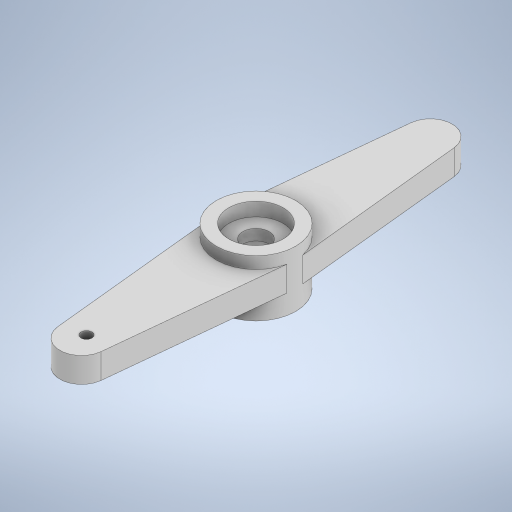
# Autodesk Inventor part: Servo_small_top
Saved by Autodesk Inventor 2023 (Build 270158000, 158)
## iProperties
Created: 2024-07-03
Part Number: Servo_small_top
Material: Generic
Document SubType Name: Modeling
Designer: Swoby
Density: 1 g/cm^3
Appearance: Default
Author: Swoby
Autodesk Inventor part; units mm, degrees
ref_plane "YZ Plane" through (0, 0, 0) normal (1, 0, 0) x (0, 1, 0)
sketch "Sketch1" plane through (0, 0, 0) normal (0, 1, 0) x (-1, 0, 0)
  circle A0 centre (0, 0) radius 2.5
  circle A1 centre (0, 0) radius 3.65
  dimension "d0" = 5
  dimension "d1" = 7.3
  constraints: 2 centre point, 2 coincident
  measures "d0" diameter of A0
  measures "d1" diameter of A1
extrude "Extrusion1" add sketch "Sketch1" along normal blind 5.2
ref_plane "Work Plane1" through (0, 3.95, 0) normal (0, 1, 0) x (1, 0, 0)
sketch "Sketch2" plane through (0, 3.95, 0) normal (0, 1, 0) x (1, 0, 0)
  circle A0 centre (0, 0) radius 2.5 projected
  circle A1 centre (0, 0) radius 1.2
  dimension "d5" = 2.4
  constraints: 1 centre point, 1 coincident
  measures "d5" diameter of A1
extrude "Extrusion2" add sketch "Sketch2" against normal blind 1
ref_plane "Work Plane2" through (0, 4.1, 0) normal (0, 1, 0) x (1, 0, 0)
sketch "Sketch3" plane through (0, 4.1, 0) normal (0, 1, 0) x (1, 0, 0)
  line L0 (5.5656, 0) -> (-5.5656, 0) construction
  circle A0 centre (0, 16.05) radius 2
  line L1 (1.9896, 16.2533) -> (3.65, 0)
  circle A1 centre (0, 0) radius 3.65 projected
  line L2 (-1.9896, 16.2533) -> (-3.65, 0)
  line L3 (0, 16.05) -> (0, 18.05)
  line L4 (0, 3.65) -> (0, -3.65) construction
  circle A2 centre (0, -16.05) radius 2
  line L5 (1.9896, -16.2533) -> (3.65, 0)
  line L6 (-1.9896, -16.2533) -> (-3.65, 0)
  line L7 (0, -16.05) -> (0, -18.05)
  point P0 (0, 0)
  point P1 (-3.5746, -0.738)
  point P2 (3.5746, -0.738)
  point P3 (-3.5746, 0.738)
  point P4 (3.5746, 0.738)
  dimension "d9" = 18.05
  dimension "d10" = 4
  constraints: 16 end point, 10 point on circle, 5 midpoint, 4 symmetric about line, 2 centre point, 2 point on line, 2 tangent, 2 vertical, 1 collinear, 1 horizontal, 1 other
  measures "d9" distance of point (0, 0) L3.end
  measures "d10" diameter of A0
extrude "Extrusion3" add sketch "Sketch3" against normal blind 2.3 contours A0 | A0 L1 A1 L2 | L5 A2 L6 A1 | A2
sketch "Sketch4" plane through (0, 4.1, 0) normal (0, 1, 0) x (1, 0, 0)
  circle A0 centre (0, -15.6) radius 0.5
  point P0 (0, 0)
  dimension "d13" = 1
  dimension "d14" = 15.6
  constraints: 1 centre point
  measures "d13" diameter of A0
  measures "d14" distance of point (0, 0) A0.centre
extrude "Extrusion4" cut sketch "Sketch4" against normal through all
body "Solid1"
